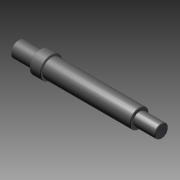
# Autodesk Inventor part: KZFC17-130-T10-P14-LA20-Q12-LB20-KC58-HC20_b
Saved by Autodesk Inventor 2011 SP1 (Build 150282100, 282)
## iProperties
Created: 2016-11-23
Part Number: KZFC17-130-T10-P14-LA20-Q12-LB20-KC58-HC20_b
Catalog Web Link: www.cadenas.de
Description: KZFN, KZFC, KZFP, KZFS, KZFF_b-Driving Shafts - One End Stepped with Shoulder -
Vendor: MISUMI
Document SubType Name: Modeling
Designer: psAdmin
Manufacturer: MISUMI
Mass: 26.2765 g
Surface Area: 72.7726 cm^2
Volume: 26.2765 cm^3
Density: 1 g/cm^3
Category: PARTsolutions
Company: MISUMI
Title: KZFC17-130-T10-P14-LA20-Q12-LB20-KC58-HC20
Author: Cadenas PARTsolutions
Comments: Driving Shafts - One End Stepped with Shoulder -
PSOL_IDENT_0: {$CADENAS_DATA\23d-libs\misumi\metric\11_rotary_shafts\11_components\kzfn\kzfn.prj},603 {VTYP=3D},{N
PSOL_IDENT_1: B=KZFC17-130-T10-P14-LA20-Q12-LB20-KC58-HC20_b},{LINA=KZFC17-130-T10-P14-LA20-Q12-LB20-KC58-HC20},{N
PSOL_IDENT_2: N=KZFN, KZFC, KZFP, KZFS, KZFF_b},{DATE=17.06.2016 05:46:52},{GEOMDATE=26.09.2014 00:00:00},{VERSION=
PSOL_IDENT_3: },{LINEID=40},{LINESUBID=-1},{WBVAR=MAT,HARD,ST,L,T,P,LA,Q,LB,ALT1,MA,MSA,MMA,ALT4,MD,MSD,MMD,ALT2,M
PSOL_IDENT_4: B,MSB,MMB,ALT5,NA,NBALT5,ALT9,KA,HAALT9,ALT10,KC,HCALT10,KD,HDALT10,ALT11,KB,HBALT11,ALT12,ZA,HAALT1
PSOL_IDENT_5: 2,AAALT12,ALT13,ZC,HCALT13,ACALT13,ZD,HDALT13,ADALT13,ALT14,ZB,HBALT14,ABALT14,ALT6,TA,TD,ALT7,TB,AL
PSOL_IDENT_6: T15,SA,ALT16,ALT17,SB,ALT18,WA,GA,AAALT18,ALT19,WD,GD,ACALT19,ALT20,WB,GB,ABALT20,ALT23}  {NB=KZFC17
PSOL_IDENT_7: -130-T10-P14-LA20-Q12-LB20-KC58-HC20_b},{LINA=KZFC17-130-T10-P14-LA20-Q12-LB20-KC58-HC20},{KT=DUMMY}
PSOL_IDENT_8: ,{PN=KZFC17-130-T10-P14-LA20-Q12-LB20-KC58-HC20},{TYPE=KZFC},{D=17},{D1=17},{MAT=S45C},{MATALG= 'S45
PSOL_IDENT_9: C','1045 Carbon Steel','SUS304','304 Stainless Steel' },{HARD=-},{HARDALG= '-','-','IHSH50','Inducti
PSOL_IDENT_10: on Hardened Surface Hardness 50HRC' },{ST=BO},{STALG= '-','-','BO','Black Oxide','ENP','Electroless
PSOL_IDENT_11: Nickel Plating'},{L=130.0},{LALG=[100:400/0.5]},{T=10},{TALG=10,15,20,25},{P=14},{PALG=[14:18/1]},{P
PSOL_IDENT_12: MIN=14},{PMAX=18},{LA=20.0},{LAALG=[5:60/0.5]},{LAMIN=5.0},{LAMAX=60.0},{Q=12},{QALG=[10:16/1]},{QMI
PSOL_IDENT_13: N=10},{QMAX=16},{LB=20.0},{LBALG=[5:45/0.5]},{LBMIN=5.0},{LBMAX=45.0},{H=20},{DSS=19},{CC=0.5},{LL=8
PSOL_IDENT_14: 0.0},{ALT1=},{ALT1ALG= '','Not applicable' },{ALT1PN=},{MA=0},{MAALG=[0]},{MAMIN=0.000},{MAMAX=0},{M
PSOL_IDENT_15: SA=0},{MSAALG=[0]},{MSAMIN=0},{MSAMAX=0},{MMA=0},{MMAALG=[0]},{MMAMIN=0},{MMAMAX=0},{MALT1=0},{APITC
PSOL_IDENT_16: H=1.00},{ALT4=},{ALT4ALG= '','w/o Shaft End D Threaded Ends','MSD','with MSD (Fine (Standard) JIS 6h
PSOL_IDENT_17: (Class 2))','MMD','with MMD (Fine (Precision) JIS 4h (Class 1))' },{ALT4PN=},{MD=0},{MDALG=[0]},{MD
PSOL_IDENT_18: MIN=0},{MDMAX=0},{MSD=0},{MSDALG=[0]},{MSDMIN=0},{MSDMAX=0},{MMD=0},{MMDALG=[0]},{MMDMIN=0},{MMDMAX=
PSOL_IDENT_19: 0},{MALT4=0},{DPITCH=1.00},{CIFMD1=0.000},{CIFMD2=15.917},{ALT2=},{ALT2ALG= '','w/o Shaft End P Thre
PSOL_IDENT_20: aded Ends','MB','with MB (Coarse JIS 6h (CLBss 2))','MSB','with MSB (Fine (Standard) JIS 6h (CLBss 2
PSOL_IDENT_21: ))','MMB','with MMB (Fine (Precision) JIS 4h (CLBss 1))' },{ALT2PN=},{MB=0},{MBALG=[0]},{MBMIN=0},{M
PSOL_IDENT_22: BMAX=0},{MSB=0},{MSBALG=[0]},{MSBMIN=0},{MSBMAX=0},{MMB=0},{MMBALG=[0]},{MMBMIN=0},{MMBMAX=0},{MALT2=
PSOL_IDENT_23: 0},{BPITCH=1.00},{ALT5=},{ALT5ALG= '','w/o Tapped Ends','NA','with NA (Tapped Left End)','NB','with
PSOL_IDENT_24: NB (Tapped Right End)','NANB','with NA + NB (Tapped Both Ends)' },{ALT5PN=},{NA=0},{NAALG= '0','N/A'
PSOL_IDENT_25: },{NAMAX=10},{NAMAX1=10},{NAMAX2=36},{NA1=0.000},{NAL=0},{NAL1=110},{PITCHA=0.00},{NBALT5=0},{NBALT
PSOL_IDENT_26: 5ALG= '0','N/A' },{NBALT5MAX=8},{NBALT5MAX1=8},{NBALT5MAX2=36},{NBALT5MAX3=36},{NBALT5MAX4=0},{NB1=0
PSOL_IDENT_27: },{NBL=0},{NBL1=110},{PITCHB=0.00},{CIFNA=0},{ALT9=},{ALT9ALG= '','w/o Shaft End P Key Groove','KA','
PSOL_IDENT_28: with KA (Shaft End P Key Groove)' },{ALT9PN=},{KA=0},{KAALG=[0]},{KAMIN=0},{KAMAX=13},{HAALT9=0},{HA
PSOL_IDENT_29: ALT9ALG=[0]},{HAALT9MIN=5},{HAALT9MAX=18},{ALT10=KC},{ALT10ALG= '','w/o Shaft End D Key Grooves','KC'
PSOL_IDENT_30: ,'with KC (Shaft End D Key Groove)','KCKD','with KC + KD (Shaft End D Two Key Grooves)' },{ALT10PN=-
PSOL_IDENT_31: KC58-HC20},{KC=58},{KCALG=[2:73/1]},{KCMIN=2},{KCMAX1=73},{KCMAX2=66},{HCALT10=20},{HCALT10ALG=[5:20
PSOL_IDENT_32: /1]},{HCALT10MIN=5},{HCALT10MAX1=20},{HCALT10MAX2=13},{KD=0},{KDALG=[0]},{KDMIN=80},{KDMAX=73},{HDAL
PSOL_IDENT_33: T10=0},{HDALT10ALG=[0]},{HDALT10MIN=5},{HDALT10MAX=78},{ALT11=},{ALT11ALG= '','w/o Shaft End Q Key G
PSOL_IDENT_34: roove','KB','with KB (Shaft End Q Key Groove)' },{ALT11PN=},{KB=0},{KBALG=[0]},{KBMIN=0},{KBMAX=14},
PSOL_IDENT_35: {HBALT11=0},{HBALT11ALG=[0]},{HBALT11MIN=4},{HBALT11MAX=18},{ALT12=},{ALT12ALG= '','w/o Shaft End P
PSOL_IDENT_36: Key Groove + Set Screw Flat','ZA','with ZA (Shaft End P Key Groove + Set Screw Flat)' },{ALT12PN=},{
PSOL_IDENT_37: ZA=0},{ZAALG=[0]},{ZAMIN=0},{ZAMAX=13},{HAALT12=0},{HAALT12ALG=[0]},{HAALT12MIN=5},{HAALT12MAX=18},{
PSOL_IDENT_38: AAALT12=0},{AAALT12ALG=[0]},{PBB=5},{PTT=3.0},{ALT13=},{ALT13ALG= '','Not applicable' },{ALT13PN=},{
PSOL_IDENT_39: ZC=0},{ZCALG=[0]},{ZCMIN=2},{ZCMAX1=73},{ZCMAX2=66},{HCALT13=0},{HCALT13ALG=[0]},{HCALT13MIN=5},{HCA
PSOL_IDENT_40: LT13MAX1=78},{HCALT13MAX2=71},{ACALT13=0},{ACALT13ALG=[0]},{ZD=0},{ZDALG=[0]},{ZDMIN=2},{ZDMAX=73},{
PSOL_IDENT_41: HDALT13=0},{HDALT13ALG=[0]},{HDALT13MIN=5},{HDALT13MAX=78},{ADALT13=0},{ADALT13ALG=[0]},{DBB=5},{DTT=
PSOL_IDENT_42: 3.0},{ALT14=},{ALT14ALG= '','w/o Shaft End Q Key Groove + Set Screw Flat','ZB','with ZB (Shaft End Q
PSOL_IDENT_43: Key Groove + Set Screw Flat)' },{ALT14PN=},{ZB=0},{ZBALG=[0]},{ZBMIN=0},{ZBMAX=14},{HBALT14=0},{HBA
PSOL_IDENT_44: LT14ALG=[0]},{HBALT14MIN=4},{HBALT14MAX=18},{ABALT14=0},{ABALT14ALG=[0]},{QBB=4},{QTT=2.5},{ALT6=},{
PSOL_IDENT_45: ALT6ALG=  '','w/o Retaining Ring Grooves','TA','with TA (Shaft End P Retaining Ring Groove)','TD','w
PSOL_IDENT_46: ith TD (Shaft End D Retaining Ring Groove)','TATD','with TA + TD (Shaft End P + Shaft End D Retainin
PSOL_IDENT_47: g Ring Grooves)' },{ALT6PN=},{TA=0},{TAALG=[0]},{TAMIN=4},{TAMAX=17},{PDD=0.0},{PMM=0.00},{TD=0},{TD
PSOL_IDENT_48: ALG=[0]},{TDMIN=4},{TDMAX=77},{DDD=0.0},{DMM=0.00},{ALT7=},{ALT7ALG=  '','w/o Retaining Ring Groove'
PSOL_IDENT_49: ,'TB','with TB (Shaft End Q Retaining Ring Groove)' },{ALT7PN=},{TB=0},{TBALG=[0]},{TBMIN=4},{TBMAX=
PSOL_IDENT_50: 17},{QDD=0.0},{QMM=0.00},{ALT15=},{ALT15ALG= '', 'w/o Shaft End P Wrench Flats', 'SA', 'with SA (Sha
PSOL_IDENT_51: ft End P Wrench Flats)' },{ALT15PN=},{SA=0},{SAALG=[0]},{SAMIN=0},{SAMAX=20},{PW1=0.0},{PLL=0},{ALT1
PSOL_IDENT_52: 6=},{ALT16ALG= '', 'w/o Shoulder Wrench Flats', 'SH', 'with SH (Shoulder Wrench Flats)' },{ALT16PN=}
PSOL_IDENT_53: ,{WALT16=0},{ALT17=},{ALT17ALG= '', 'w/o Shaft End Q Wrench Flats', 'SB', 'with SB (Shaft End Q Wren
PSOL_IDENT_54: ch Flats)' },{ALT17PN=},{SB=0},{SBALG=[0]},{SBMIN=0},{SBMAX=20},{QW1=0.0},{QLL=0},{ALT18=},{ALT18ALG=
PSOL_IDENT_55: '','w/o Shaft End P 2 Set Screw Flats (Angle Specified)','WA','with WA (Shaft End P 2 Set Screw Fla
PSOL_IDENT_56: ts (Angle Specified))' },{ALT18PN=},{WA=0},{WAALG=[0]},{WAMIN=0},{WAMAX=17},{GA=0},{GAALG=[0]},{GAMI
PSOL_IDENT_57: N=3},{GAMAX=20},{AAALT18=0},{AAALT18ALG=[0]},{PH=0.0},{ALT19=},{ALT19ALG= '','w/o Shaft End D 2 Set
PSOL_IDENT_58: Screw Flats (Angle Specified)','WD','with WD (Shaft End D 2 Set Screw Flats (Angle Specified))' },{A
PSOL_IDENT_59: LT19PN=},{WD=0},{WDALG=[0]},{WDMIN=2},{WDMAX=77},{GD=0},{GDALG=[0]},{GDMIN=3},{GDMAX=80},{ACALT19=0}
PSOL_IDENT_60: ,{ACALT19ALG=[0]},{DH=0.0},{ALT20=},{ALT20ALG= '','w/o Shaft End Q 2 Set Screw Flats (Angle Specifie
PSOL_IDENT_61: d)','WB','with WB (Shaft End Q 2 Set Screw Flats (Angle Specified))' },{ALT20PN=},{WB=0},{WBALG=[0]}
PSOL_IDENT_62: ,{WBMIN=0},{WBMAX=17},{GB=0},{GBALG=[0]},{GBMIN=3},{GBMAX=20},{ABALT20=0},{ABALT20ALG=[0]},{QH=0.0},
PSOL_IDENT_63: {ALT23=},{ALT23PN=},{ERRORPN=},{ERRORPALT16=OK},{ERRORALT15=OK},{ERRORALT16=OK},{ERRORALT115=OK},{ER
PSOL_IDENT_64: RORALT118=OK},{ERRORALT25=OK},{ERRORALT27=OK},{ERRORALT217=OK},{ERRORALT220=OK},{ERRORALT45=OK},{ERR
PSOL_IDENT_65: ORALT46=OK},{ERRORALT419=OK},{ERRORALT59=OK},{ERRORALT510=OK},{ERRORALT511=OK},{ERRORALT512=OK},{ERR
PSOL_IDENT_66: ORALT513=OK},{ERRORALT514=OK},{ERRORALT515=OK},{ERRORALT516=},{ERRORALT517=OK},{ERRORALT518=OK},{ERR
PSOL_IDENT_67: ORALT519=OK},{ERRORALT520=OK},{ERRORALT69=OK},{ERRORALT610=OK},{ERRORALT612=OK},{ERRORALT613=OK},{ER
PSOL_IDENT_68: RORALT615=OK},{ERRORALT618=OK},{ERRORALT619=OK},{ERRORALT711=OK},{ERRORALT714=OK},{ERRORALT717=OK},{
PSOL_IDENT_69: ERRORALT720=OK},{ERRORALT915=OK},{ERRORALT918=OK},{ERRORALT1019=OK},{ERRORALT1117=OK},{ERRORALT1120=
PSOL_IDENT_70: OK},{ERRORALT1215=OK},{ERRORALT1417=OK},{ERRORALT1518=OK},{ERRORALT1720=OK}
NN: KZFN, KZFC, KZFP, KZFS, KZFF_b
NT: Driving Shafts - One End Stepped with Shoulder -
NB: KZFC17-130-T10-P14-LA20-Q12-LB20-KC58-HC20_b
NBSYN: $PN._b
LINA: KZFC17-130-T10-P14-LA20-Q12-LB20-KC58-HC20
PN: KZFC17-130-T10-P14-LA20-Q12-LB20-KC58-HC20
D: 17
MAT: 1045 Carbon Steel
HARD: -
ST: Black Oxide
L: 130.0
T: 10
P: 14
LA: 20.0
Q: 12
LB: 20.0
H: 20
DSS: 19
ALT1: Not applicable
MA: 0
MSA: 0
MMA: 0
ALT4: w/o Shaft End D Threaded Ends
MD: 0
MSD: 0
MMD: 0
ALT2: w/o Shaft End P Threaded Ends
MB: 0
MSB: 0
MMB: 0
ALT5: w/o Tapped Ends
NA: N/A
NBALT5: N/A
ALT9: w/o Shaft End P Key Groove
KA: 0
HAALT9: 0
ALT10: with KC (Shaft End D Key Groove)
KC: 58
HCALT10: 20
KD: 0
HDALT10: 0
ALT11: w/o Shaft End Q Key Groove
KB: 0
HBALT11: 0
ALT12: w/o Shaft End P Key Groove + Set Screw Flat
ZA: 0
HAALT12: 0
AAALT12: 0
ALT13: Not applicable
ZC: 0
HCALT13: 0
ACALT13: 0
ZD: 0
HDALT13: 0
ADALT13: 0
ALT14: w/o Shaft End Q Key Groove + Set Screw Flat
ZB: 0
HBALT14: 0
ABALT14: 0
ALT6: w/o Retaining Ring Grooves
TA: 0
PDD: 0.0
PMM: 0.00
TD: 0
DDD: 0.0
DMM: 0.00
ALT7: w/o Retaining Ring Groove
TB: 0
QDD: 0.0
QMM: 0.00
ALT15: w/o Shaft End P Wrench Flats
SA: 0
PW1: 0.0
PLL: 0
ALT16: w/o Shoulder Wrench Flats
ALT17: w/o Shaft End Q Wrench Flats
SB: 0
QW1: 0.0
QLL: 0
ALT18: w/o Shaft End P 2 Set Screw Flats (Angle Specified)
WA: 0
GA: 0
AAALT18: 0
PH: 0.0
ALT19: w/o Shaft End D 2 Set Screw Flats (Angle Specified)
WD: 0
GD: 0
ACALT19: 0
DH: 0.0
ALT20: w/o Shaft End Q 2 Set Screw Flats (Angle Specified)
WB: 0
GB: 0
ABALT20: 0
QH: 0.0
ALT23: w/o D Tolerance Change
SUPPLIER: MISUMI
ARTICLENO: KZFC17-130-T10-P14-LA20-Q12-LB20-KC58-HC20_b
BOMINFO: KZFC17-130-T10-P14-LA20-Q12-LB20-KC58-HC20
CREATOR: CADENAS GmbH
Autodesk Inventor part; units mm, degrees
ref_plane "YZ Plane" through (0, 0, 0) normal (1, 0, 0) x (0, 1, 0)
ref_plane "XZ Plane" through (0, 0, 0) normal (0, 1, 0) x (-1, 0, 0)
ref_plane "XY Plane" through (0, 0, 0) normal (0, 0, 1) x (1, 0, 0)
sketch "Sketch_1" plane through (0, 0, 0) normal (0, 0, 1) x (1, 0, 0)
  line L0 (130, 0) -> (0, 0)
  line L1 (0, 0) -> (0, 6.5)
  line L2 (0, 6.5) -> (0.5, 7)
  line L3 (0.5, 7) -> (20, 7)
  line L4 (20, 7) -> (20, 9.5)
  line L5 (20, 9.5) -> (20.5, 10)
  line L6 (20.5, 10) -> (29.5, 10)
  line L7 (29.5, 10) -> (30, 9.5)
  line L8 (30, 9.5) -> (30, 8.5)
  line L9 (30, 8.5) -> (109.5, 8.5)
  line L10 (109.5, 8.5) -> (110, 8)
  line L11 (110, 8) -> (110, 6)
  line L12 (110, 6) -> (129.5, 6)
  line L13 (129.5, 6) -> (130, 5.5)
  line L14 (130, 5.5) -> (130, 0)
  line L15 (130, 0) -> (0, 0)
  constraints: 32 end point
revolve "Revolution1" add sketch "Sketch_1" angle 360 about axis through (130, 0, 0) along (1, 0, 0)
sketch "Sketch_2" plane through (0, 0, 0) normal (0, 0, 1) x (1, 0, 0)
  line L0 (50, 0) -> (-50, 0)
  line L1 (18.5, 6.7) -> (20, 6.7)
  line L2 (20, 6.7) -> (20, 20.7)
  line L3 (20, 20.7) -> (18.5, 20.7)
  line L4 (18.5, 20.7) -> (18.5, 6.7)
  constraints: 10 end point
revolve "Revolution2" cut sketch "Sketch_2" angle 360 about axis through (50, 0, 0) along (1, 0, 0)
sketch "Sketch_3" plane through (0, 0, 0) normal (0, 0, 1) x (1, 0, 0)
  line L0 (260, 0) -> (-260, 0)
  line L1 (30, 8.2) -> (31.5, 8.2)
  line L2 (31.5, 8.2) -> (31.5, 22.2)
  line L3 (31.5, 22.2) -> (30, 22.2)
  line L4 (30, 22.2) -> (30, 8.2)
  constraints: 10 end point
revolve "Revolution3" cut sketch "Sketch_3" angle 360 about axis through (260, 0, 0) along (1, 0, 0)
sketch "Sketch_4" plane through (0, 0, 0) normal (0, 0, 1) x (1, 0, 0)
  line L0 (50, 0) -> (-50, 0)
  line L1 (110, 5.7) -> (111.5, 5.7)
  line L2 (111.5, 5.7) -> (111.5, 19.7)
  line L3 (111.5, 19.7) -> (110, 19.7)
  line L4 (110, 19.7) -> (110, 5.7)
  constraints: 10 end point
revolve "Revolution4" cut sketch "Sketch_4" angle 360 about axis through (50, 0, 0) along (1, 0, 0)
sketch "Sketch_15" plane through (0, 8.5, 0) normal (0, 1, 0) x (1, 0, 0)
  arc A0 (34.5, 2.5) -> (34.5, -2.5) centre (34.5, 0) ccw
  line L0 (34.5, -2.5) -> (49.5, -2.5)
  arc A1 (49.5, -2.5) -> (49.5, 2.5) centre (49.5, 0) ccw
  line L1 (49.5, 2.5) -> (34.5, 2.5)
  constraints: 4 end point, 4 point on circle, 2 centre point
extrude "Extrusion1" cut sketch "Sketch_15" against normal blind 3
body "Solid1"
